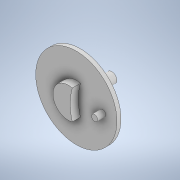
# Autodesk Inventor part: driverwheel
Saved by Autodesk Inventor 2022 (Build 260153000, 153)
## iProperties
Created: 2023-01-29
Part Number: driverwheel
Material: Generic
Document SubType Name: Modeling
Designer: karee
Density: 1 g/cm^3
Appearance: Default
Author: karee
Autodesk Inventor part; units mm, degrees
ref_plane "YZ Plane" through (0, 0, 0) normal (1, 0, 0) x (0, 1, 0)
ref_plane "XZ Plane" through (0, 0, 0) normal (0, 1, 0) x (-1, 0, 0)
ref_plane "XY Plane" through (0, 0, 0) normal (0, 0, 1) x (1, 0, 0)
sketch "Sketch1" plane through (0, 0, 0) normal (0, 0, 1) x (1, 0, 0)
  circle A0 centre (0, 0) radius 40
  dimension "d0" = 40
  constraints: 1 centre point, 1 coincident
  measures "d0" radius of A0
extrude "Extrusion1" add sketch "Sketch1" along normal blind 4
sketch "Sketch2" plane through (0, 0, 4) normal (0, 0, 1) x (1, 0, 0)
  arc A0 (4.0325, 14.4478) -> (4.0325, -14.4478) centre (0, 0) ccw
  arc A1 (4.0325, 14.4478) -> (4.0325, -14.4478) centre (54.3652, 0) ccw
  dimension "d3" = 15
  constraints: 4 point on circle, 2 centre point, 1 coincident
  measures "d3" radius of A0
extrude "Extrusion2" add sketch "Sketch2" along normal blind 8
sketch "Sketch3" plane through (0, 0, 4) normal (0, 0, 1) x (1, 0, 0)
  circle A0 centre (26, 0) radius 3
  point P0 (0, 0)
  dimension "d6" = 3
  constraints: 1 centre point
  measures "d6" radius of A0
sketch "Sketch4" plane through (0, 0, 0) normal (0, 0, -1) x (-1, 0, 0)
  circle A0 centre (0, 0) radius 10
  dimension "d9" = 10
  constraints: 1 centre point, 1 coincident
  measures "d9" radius of A0
extrude "Extrusion4" add sketch "Sketch4" along normal blind 6
sketch "Sketch5" plane through (0, 0, -6) normal (0, 0, -1) x (-1, 0, 0)
  circle A0 centre (0, 0) radius 5
  circle A1 centre (0, 0) radius 3
  dimension "d12" = 5
  dimension "d13" = 3
  constraints: 2 centre point, 2 coincident
  measures "d12" radius of A0
  measures "d13" radius of A1
extrude "Extrusion5" add sketch "Sketch5" along normal blind 25
sketch "Sketch6" plane through (0, 0, 0) normal (0, 1, 0) x (-1, 0, 0)
  circle A0 centre (0, -21) radius 2
  point P0 (0, 0)
  dimension "d16" = 2
  constraints: 1 centre point
  measures "d16" radius of A0
extrude "Extrusion6" cut sketch "Sketch6" along normal mid plane 25
extrude "Extrusion7" add sketch "Sketch3" along normal blind 8
body "Solid1"
